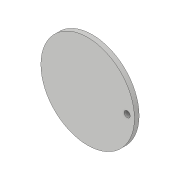
# Autodesk Inventor part: FLAPPER
Saved by Autodesk Inventor 2019 (Build 230136000, 136)
## iProperties
Created: 2019-10-17
Part Number: FLAPPER
Material: Generic
Document SubType Name: Modeling
Designer: Admin
Density: 1 g/cm^3
Appearance: Default
Author: Admin
Autodesk Inventor part; units mm, degrees
ref_plane "YZ Plane" through (0, 0, 0) normal (1, 0, 0) x (0, 1, 0)
ref_plane "XZ Plane" through (0, 0, 0) normal (0, 1, 0) x (-1, 0, 0)
ref_plane "XY Plane" through (0, 0, 0) normal (0, 0, 1) x (1, 0, 0)
sketch "Sketch1" plane through (0, 0, 0) normal (0, 0, 1) x (1, 0, 0)
  circle A0 centre (0, 0) radius 20
  dimension "d0" = 40
  constraints: 1 centre point, 1 coincident
  measures "d0" diameter of A0
extrude "Extrusion1" add sketch "Sketch1" along normal blind 2
sketch "Sketch2" plane through (0, 0, 2) normal (0, 0, 1) x (1, 0, 0)
  line L0 (19.8968, 0) -> (16.8968, 0)
  circle A0 centre (16.8968, 0) radius 1.3
  point P0 (0, 0)
  dimension "d3" = 3
  dimension "d4" = 2.6
  constraints: 2 end point, 1 centre point, 1 coincident, 1 horizontal
  measures "d3" distance of L0.start L0.end
  measures "d4" diameter of A0
extrude "Extrusion2" cut sketch "Sketch2" against normal blind 2
body "Solid1"
